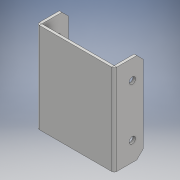
# Autodesk Inventor part: 4-4
Saved by Autodesk Inventor 2017 (Build 210142000, 142)
## iProperties
Part Number: 4-4
Material: 一般
Document SubType Name: 板金
Designer: Brian
Density: 1 g/cm^3
Sheet Metal Rule: 預設
Appearance: 預設
Author: Brian
Autodesk Inventor part; units mm, degrees
ref_plane "YZ Plane" through (0, 0, 0) normal (1, 0, 0) x (0, 1, 0)
ref_plane "XZ Plane" through (0, 0, 0) normal (0, 1, 0) x (-1, 0, 0)
ref_plane "XY Plane" through (0, 0, 0) normal (0, 0, 1) x (1, 0, 0)
sketch "草圖1" plane through (0, 0, 0) normal (0, 1, 0) x (-1, 0, 0)
  line L0 (0, 0) -> (-60, 0)
  line L1 (-60, 0) -> (-60, -70)
  line L2 (-60, -70) -> (0, -70)
  line L3 (0, -70) -> (0, 0)
  dimension "d0" = 60
  dimension "d1" = 70
  measures "d0" distance of L1.end L2.end
  measures "d1" distance of L2.end L0.start
extrude "平板1" add sketch "草圖1" along normal blind 2
sketch "草圖2" plane through (2, 0, 0) normal (-1, 0, 0) x (0, -1, 0)
  line L0 (0, -70) -> (0, 0)
  line L1 (0, 0) -> (-22.5, 0)
  line L2 (-22.5, 0) -> (-22.5, -70)
  line L3 (-22.5, -70) -> (0, -70)
  constraints: 6 end point, 1 horizontal, 1 perpendicular, 1 vertical
edge flange "凸緣1" height 22.5 angle 90 thickness 2 bend radius 0 thickness toward (-1, 0, 0) relief tear relief width 2 relief depth 1 edges at (0, 2, -35) wall of the first edge with corners at (2, 0, -70) (2, 0, 0) (2, 22.5, 0) (2, 22.5, -70)
bend "折彎1"
corner "轉角1"
sketch "草圖3" plane through (58, 0, -70) normal (1, 0, 0) x (0, 1, 0)
  line L0 (0, 70) -> (0, 0)
  line L1 (0, 0) -> (22.5, 0)
  line L2 (22.5, 0) -> (22.5, 70)
  line L3 (22.5, 70) -> (0, 70)
  constraints: 6 end point, 1 horizontal, 1 perpendicular, 1 vertical
edge flange "凸緣2" height 22.5 angle 90 thickness 2 bend radius 0 thickness toward (1, 0, 0) relief tear relief width 2 relief depth 1 edges at (60, 2, -35) wall of the first edge with corners at (58, 0, 0) (58, 0, -70) (58, 22.5, -70) (58, 22.5, 0)
bend "折彎2"
corner "轉角2"
chamfer "轉角倒角1" distance 5 angle 45 4 edges at (1, 22.5, 0) (1, 22.5, -70) (59, 22.5, 0) (59, 22.5, -70)
sketch "草圖4" plane through (60, 2.001, 0) normal (1, 0, 0) x (0, 0, -1)
  line L0 (15, 11.999) -> (55, 11.999)
  line L1 (70, -2.001) -> (0, -2.001) projected
  line L2 (0, 0) -> (0, 15.499) projected
  dimension "d26" = 40
  dimension "d27" = 14
  dimension "d28" = 15
  constraints: 2 end point, 1 horizontal
  measures "d26" distance of L0.start L0.end
  measures "d27" distance between parallel lines of L1 L0
  measures "d28" distance from line of L2 L0.start
hole "孔1" at (60, 14, -15) at (60, 14, -55) direction (-1, 0, 0) diameter 5 depth 80 tip angle 118
equation "\"d3\" = 折彎離隙寬度"
equation "\"d4\" = 折彎離隙深度"
equation "\"d5\" = 最小剩餘"
equation "\"d6\" = 折彎半徑"
equation "\"d10\" = 轉角離隙大小"
equation "\"d11\" = 間隙大小"
equation "\"d12\" = Jacobi半徑大小"
equation "\"d13\" = 折彎離隙寬度"
equation "\"d14\" = 折彎離隙深度"
equation "\"d15\" = 最小剩餘"
equation "\"d16\" = 折彎半徑"
equation "\"d20\" = 轉角離隙大小"
equation "\"d21\" = 間隙大小"
equation "\"d22\" = Jacobi半徑大小"
equation "\"折彎半徑\" = 厚度"
equation "\"折彎離隙寬度\" = 厚度"
equation "\"折彎離隙深度\" = 0.5 * 厚度"
equation "\"轉角離隙大小\" = 4 * 厚度"
equation "\"最小剩餘\" = 2 * 厚度"
equation "\"轉移半徑\" = 折彎半徑"
equation "\"Jacobi半徑大小\" = 厚度"
equation "\"間隙大小\" = 厚度"
equation "\"d2\" = 折彎半徑"
equation "\"厚度\" = 2"
